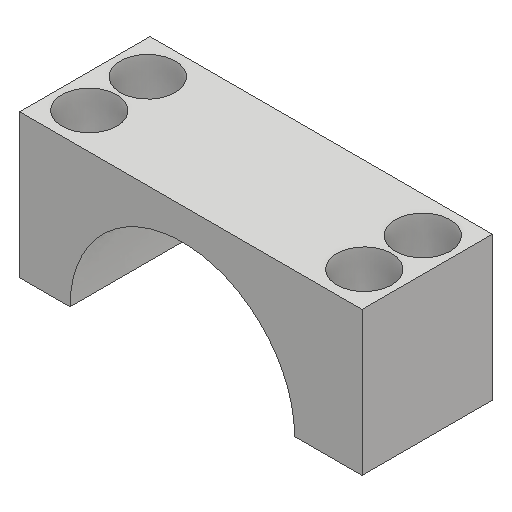
# Autodesk Inventor part: 3DP_PLA_Motor_mounting_bracket_front
Saved by Autodesk Inventor 2025 (Build 290162010, 162A)
## iProperties
Created: 2016-05-01
Part Number: 3DP_PLA_Motor_mounting_bracket_front
Material: Ogólny
Document SubType Name: Modeling
Designer: Andrzej
Density: 1 g/cm^3
Appearance: Domyślna
Mass: 4.33086 g
Surface Area: 32.703 cm^2
Volume: 4.33086 cm^3
Author: Andrzej
Autodesk Inventor part; units mm, degrees
ref_plane "YZ Plane" through (0, 0, 0) normal (1, 0, 0) x (0, 1, 0)
ref_plane "XZ Plane" through (0, 0, 0) normal (0, 1, 0) x (-1, 0, 0)
ref_plane "XY Plane" through (0, 0, 0) normal (0, 0, 1) x (1, 0, 0)
sketch "Szkic1" plane through (0, 0, 0) normal (0, 0, 1) x (1, 0, 0)
  line L0 (-23.252, 12.6301) -> (16.748, 12.6301)
  line L1 (16.748, 12.6301) -> (16.748, -1.8699)
  line L2 (16.748, -1.8699) -> (-23.252, -1.8699)
  line L3 (-23.252, -1.8699) -> (-23.252, 12.6301)
  point P0 (0, 0)
  dimension "d0" = 40
  dimension "d1" = 14.5
  constraints: 8 end point, 2 parallel, 1 horizontal, 1 perpendicular
  measures "d0" distance of L1.end L2.end
  measures "d1" distance of L0.end L1.end
extrude "Wyciągnięcie proste1" add sketch "Szkic1" along normal blind 16
sketch "Szkic2" plane through (-23.252, -1.8699, 0) normal (0, -1, 0) x (1, 0, 0)
  line L0 (40, 0) -> (40, 16) projected
  line L1 (0, 0) -> (0, 16) projected
  circle A0 centre (20, 0) radius 12.5
  point P0 (23.252, 0)
  dimension "d4" = 40
  dimension "d5" = 20
  dimension "d6" = 25
  constraints: 1 centre point, 1 coincident
  measures "d4" distance between parallel lines of L0 L1
  measures "d5" distance from line of L1 point (20, 0)
  measures "d6" diameter of A0
extrude "Wyciągnięcie proste2" cut sketch "Szkic2" against normal blind 17
sketch "Szkic3" plane through (0, 0, 0) normal (0, 0, -1) x (-1, 0, 0)
  line L0 (15.752, 12.6301) -> (15.752, -1.8699) projected
  line L1 (15.752, -1.8699) -> (23.252, -1.8699) projected
  line L2 (23.252, -1.8699) -> (23.252, 12.6301) projected
  line L3 (23.252, 12.6301) -> (15.752, 12.6301) projected
  line L4 (-9.248, -1.8699) -> (-9.248, 12.6301) projected
  line L5 (-9.248, 12.6301) -> (-16.748, 12.6301) projected
  line L6 (-16.748, 12.6301) -> (-16.748, -1.8699) projected
  line L7 (-16.748, -1.8699) -> (-9.248, -1.8699) projected
  point P0 (0, 0)
  point P1 (17.602, 2.1301)
  point P2 (17.602, 8.6301)
  point P3 (-12.998, 2.1301)
  point P4 (-12.998, 8.6301)
  dimension "d9" = 5.65
  dimension "d10" = 5.65
  dimension "d11" = 3.75
  dimension "d12" = 3.75
  dimension "d13" = 4
  dimension "d14" = 4
  dimension "d15" = 6.5
  dimension "d16" = 6.5
  dimension "d34" = 14.5
  measures "d9" distance from line of L2 point (17.602, 2.13)
  measures "d10" distance from line of L2 point (17.602, 8.63)
  measures "d11" distance from line of L6 point (-12.998, 8.63)
  measures "d12" distance from line of L6 point (-12.998, 2.13)
  measures "d13" distance from line of L1 point (17.602, 2.13)
  measures "d14" distance from line of L7 point (-12.998, 2.13)
  measures "d15" distance of point (17.602, 8.63) point (17.602, 2.13)
  measures "d16" distance of point (-12.998, 2.13) point (-12.998, 8.63)
  measures "d34" distance of L1.end L2.end
hole "Otwór1" at (-17.602, 2.1301, 0) at (-17.602, 8.6301, 0) at (12.998, 2.1301, 0) at (12.998, 8.6301, 0) direction (0, 0, 1) diameter 3.25 end through all
sketch "Szkic5" plane through (0, 0, 16) normal (0, 0, 1) x (1, 0, 0)
  circle A0 centre (12.998, 2.1301) radius 1.625 projected
  circle A1 centre (-17.602, 2.1301) radius 1.625 projected
  circle A2 centre (-17.602, 8.6301) radius 1.625 projected
  circle A3 centre (12.998, 8.6301) radius 1.625 projected
  line L0 (16.748, 12.6301) -> (-23.252, 12.6301) projected
  line L1 (-23.252, 12.6301) -> (-23.252, -1.8699) projected
  line L2 (-23.252, -1.8699) -> (16.748, -1.8699) projected
  line L3 (16.748, -1.8699) -> (16.748, 12.6301) projected
  point P0 (0, 0)
  constraints: 4 coincident
hole "Otwór2" at (-17.602, 2.1301, 16) at (-17.602, 8.6301, 16) at (12.998, 8.6301, 16) at (12.998, 2.1301, 16) direction (0, 0, -1) diameter 6.1 depth 5
sketch "Szkic7" plane through (-23.252, -1.8699, 0) normal (-1, 0, 0) x (0, 0, 1)
  line L0 (0, 0) -> (0, 14.5) projected
  line L1 (0, 0) -> (16, 0) projected
  line L2 (16, 14.5) -> (16, 0) projected
  line L3 (0, 14.5) -> (16, 14.5) projected
  point P0 (0, 1.8699)
extrude "Wyciągnięcie proste4" cut sketch "Szkic7" against normal blind 1.9
equation "\"d5\" = 0.5 * d4"
equation "\"d13\" = -0.5 * d15 + 0.5 * d34"
equation "\"d14\" = d13"
equation "\"d16\" = d15"
